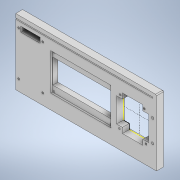
# Autodesk Inventor part: 2020-04-12 CubeBaseFull
Saved by Autodesk Inventor 2020 (Build 240168000, 168)
## iProperties
Created: 2019-12-01
Part Number: 2020-04-12 CubeBaseFull
Material: Generic
Document SubType Name: Modeling
Designer: torto
Density: 1 g/cm^3
Appearance: Default
length: 230.251 mm
height: 107.950 mm
d3: 6.350 mm
d4: 6.350 mm
d5: 223.901 mm
d6: 1.524 mm
spacing: 35.983 mm
d9: 6.350 mm
d10: 3.500 mm
d11: 2.000 ul
d13: 35.983 mm
thickness: 12.700 mm
d19: 0.00 deg
d21: 6.350 mm
d22: 6.350 mm
d23: 223.901 mm
d24: 1.524 mm
d25: 6.350 mm
d26: 0.00 deg
d33: 6.350 mm
d34: 35.983 mm
ScrewDiameter: 4.000 mm
d36: 6.350 mm
d37: 35.983 mm
d38: 4.000 mm
d39: 12.700 mm
d40: 0.00 deg
d49: 106.626 mm
d50: 53.975 mm
LcdLength: 97.300 mm
LcdHeight: 39.800 mm
LcdBorderHeight: 60.200 mm
LcdBorderLength: 98.300 mm
d66: 9.900 mm
d67: 0.00 deg
LcdPcbThickness: 2.800 mm
d69: 0.00 deg
LcdFrameHoleOffset: 2.500 mm
d71: 2.500 mm
LcdFrameHoleDiameter: 3.000 mm
LcdScrewDepth: 6.000 mm
d74: 0.00 deg
InputHeight: 57.400 mm
InputLength: 52.500 mm
InputThickness: 1.600 mm
d78: 0.00 deg
InputHoleSpacing: 0.172 in
d80: 0.278 in
InputScrewDiameter: 3.500 mm
d82: 14.100 mm
d83: 8.500 mm
d84: 11.100 mm
d85: 0.00 deg
InputHoleSpacingX: 7.100 mm
InputHoleSpacingY: 4.250 mm
ScrewDiameterUntapped: 4.000 mm
ScrewCapDiameter: 3.500 mm
PcbThickness: 1.651 mm
TopScrewDiameter: 4.000 mm
InputScrewDiameterUntapped: 2.500 mm
InputScrewDiameterFull: 3.500 mm
InputCornerLengthX: 9.500 mm
InputCornerLengthY: 8.700 mm
UpperInputHoleSpacingY: 4.350 mm
LeftInputHoleSpacingX: 7.100 mm
NWInputHoleSpacingX: 7.250 mm
LcdFrameHoleDiameterUntapped: 2.500 mm
Author: torto
Autodesk Inventor part; units mm, degrees
ref_plane "YZ Plane" through (0, 0, 0) normal (1, 0, 0) x (0, 1, 0)
ref_plane "XZ Plane" through (0, 0, 0) normal (0, 1, 0) x (-1, 0, 0)
ref_plane "XY Plane" through (0, 0, 0) normal (0, 0, 1) x (1, 0, 0)
sketch "Sketch1" plane through (0, 0, 0) normal (0, 0, 1) x (1, 0, 0)
  line L0 (0, 0) -> (230.251, 0)
  line L1 (230.251, 0) -> (230.251, 107.95)
  line L2 (230.251, 107.95) -> (0, 107.95)
  line L3 (0, 107.95) -> (0, 0)
  line L4 (230.251, 107.95) -> (223.901, 107.95) construction
  line L5 (223.901, 107.95) -> (223.901, 101.6) construction
  line L6 (223.901, 101.6) -> (230.251, 101.6) construction
  line L7 (230.251, 101.6) -> (230.251, 107.95) construction
  line L8 (223.901, 101.6) -> (0, 101.6)
  line L9 (0, 101.6) -> (0, 100.076)
  line L10 (0, 100.076) -> (223.901, 100.076)
  line L11 (223.901, 100.076) -> (223.901, 101.6)
  line L12 (230.251, 0) -> (223.901, 0) construction
  line L13 (223.901, 0) -> (223.901, 35.9833) construction
  line L14 (223.901, 35.9833) -> (230.251, 35.9833) construction
  line L15 (230.251, 35.9833) -> (230.251, 0) construction
  circle A0 centre (223.901, 35.9833) radius 2
  circle A1 centre (223.901, 71.9667) radius 2
  dimension "length" = 230.251
  dimension "height" = 107.95
  dimension "d3" = 6.35
  dimension "d4" = 6.35
  dimension "d5" = 223.901
  dimension "d6" = 1.524
  dimension "spacing" = 35.9833
  dimension "d9" = 6.35
  dimension "TopScrewDiameter" = 4
  dimension "d13" = 35.9833
  constraints: 32 end point, 8 parallel, 4 horizontal, 4 perpendicular, 2 centre point, 2 coincident, 1 vertical, 3 other
  measures "length" distance of L2.end L1.end
  measures "height" distance of L1.end L0.end
  measures "d3" distance of L5.end L4.end
  measures "d4" distance of L5.end L6.end
  measures "d5" distance of L10.end L9.end
  measures "d6" distance of L9.end L8.end
  measures "spacing" distance of L12.end L13.end
  measures "d9" distance of L13.end L14.end
  measures "TopScrewDiameter" diameter of A0
  measures "d13" distance of A0.centre A1.centre
extrude "Generic Shape" add sketch "Sketch1" along normal blind 12.7
chamfer "Chamfer Outside Edges" distance 1.5 angle 45 3 edges at (115.1255, 107.95, 0) (230.251, 107.95, 6.35) (230.251, 53.975, 0)
sketch "ScrewCapDiameter" plane through (0, 0, 0) normal (0, 0, -1) x (-1, 0, 0)
  circle A0 centre (-223.901, 71.9667) radius 2 projected
  circle A1 centre (-223.901, 71.9667) radius 4
  circle A2 centre (-223.901, 35.9833) radius 2 projected
  circle A3 centre (-223.901, 35.9833) radius 4
  point P0 (0, 0)
  dimension "d106" = 8
  dimension "d107" = 8
  constraints: 2 centre point, 2 coincident
  measures "d106" diameter of A1
  measures "d107" diameter of A3
extrude "ScrewCapCountersink" cut sketch "ScrewCapDiameter" against normal blind 4
sketch "PcbNotchDimensions" plane through (0, 0, 12.7) normal (0, 0, 1) x (1, 0, 0)
  line L0 (230.251, 107.95) -> (0, 107.95) construction
  line L1 (230.251, 107.95) -> (223.901, 107.95) construction
  line L2 (223.901, 107.95) -> (223.901, 101.6) construction
  line L3 (223.901, 101.6) -> (230.251, 101.6) construction
  line L4 (230.251, 101.6) -> (230.251, 107.95) construction
  line L5 (223.901, 101.6) -> (0, 101.6)
  line L6 (0, 101.6) -> (0, 99.949)
  line L7 (0, 99.949) -> (223.901, 99.949)
  line L8 (223.901, 99.949) -> (223.901, 101.6)
  point P0 (0, 0)
  dimension "d21" = 6.35
  dimension "d22" = 6.35
  dimension "d23" = 223.901
  dimension "PcbThickness" = 1.651
  constraints: 16 end point, 4 parallel, 2 horizontal, 2 perpendicular
  measures "d21" distance of L2.end L1.end
  measures "d22" distance of L2.end L3.end
  measures "d23" distance of L7.end L6.end
  measures "PcbThickness" distance of L6.end L5.end
extrude "PCB Notch" cut sketch "PcbNotchDimensions" against normal blind 6.35
sketch "UntappedScrewHoleDimensions" plane through (0, 0, 0) normal (-1, 0, 0) x (0, 0, 1)
  line L0 (0, 0) -> (6.35, 0) construction
  line L1 (6.35, 0) -> (6.35, 35.9833) construction
  line L2 (6.35, 35.9833) -> (0, 35.9833) construction
  line L3 (0, 35.9833) -> (0, 0) construction
  circle A0 centre (6.35, 35.9833) radius 2
  line L4 (0, 107.95) -> (6.35, 107.95) construction
  line L5 (6.35, 107.95) -> (6.35, 71.9667) construction
  line L6 (6.35, 71.9667) -> (0, 71.9667) construction
  line L7 (0, 71.9667) -> (0, 107.95) construction
  circle A1 centre (6.35, 71.9667) radius 2
  dimension "d33" = 6.35
  dimension "d34" = 35.9833
  dimension "ScrewDiameterUntapped" = 4
  dimension "d36" = 6.35
  dimension "d37" = 35.9833
  dimension "d38" = 4
  constraints: 16 end point, 4 parallel, 2 centre point, 2 coincident, 2 horizontal, 2 perpendicular
  measures "d33" distance of L2.end L1.end
  measures "d34" distance of L1.end L0.end
  measures "ScrewDiameterUntapped" diameter of A0
  measures "d36" distance of L5.end L6.end
  measures "d37" distance of L4.end L5.end
  measures "d38" diameter of A1
extrude "UntappedScrewDepth" cut sketch "UntappedScrewHoleDimensions" against normal blind 12.7
sketch "LCD" plane through (0, 0, 0) normal (0, 0, -1) x (-1, 0, 0)
  line L0 (0, 0) -> (-230.251, 0) construction
  line L1 (0, 0) -> (-106.6255, 0) construction
  line L2 (-106.6255, 0) -> (-106.6255, 53.975) construction
  line L3 (-106.6255, 53.975) -> (0, 53.975) construction
  line L4 (0, 53.975) -> (0, 0) construction
  line L5 (-155.2755, 73.875) -> (-57.9755, 73.875)
  line L6 (-57.9755, 73.875) -> (-57.9755, 34.075)
  line L7 (-57.9755, 34.075) -> (-155.2755, 34.075)
  line L8 (-155.2755, 34.075) -> (-155.2755, 73.875)
  line L9 (-155.2755, 73.875) -> (-57.9755, 34.075) construction
  line L10 (-57.9755, 73.875) -> (-155.2755, 34.075) construction
  line L11 (-155.7755, 84.075) -> (-57.4755, 84.075)
  line L12 (-57.4755, 84.075) -> (-57.4755, 23.875)
  line L13 (-57.4755, 23.875) -> (-155.7755, 23.875)
  line L14 (-155.7755, 23.875) -> (-155.7755, 84.075)
  line L15 (-155.7755, 84.075) -> (-57.4755, 23.875) construction
  line L16 (-57.4755, 84.075) -> (-155.7755, 23.875) construction
  dimension "d49" = 106.6255
  dimension "d50" = 53.975
  dimension "LcdLength" = 97.3
  dimension "LcdHeight" = 39.8
  dimension "LcdBorderHeight" = 60.2
  dimension "LcdBorderLength" = 98.3
  constraints: 32 end point, 6 parallel, 4 midpoint, 3 horizontal, 3 perpendicular
  measures "d49" distance of L2.end L3.end
  measures "d50" distance of L1.end L2.end
  measures "LcdLength" distance of L6.end L7.end
  measures "LcdHeight" distance of L7.end L5.start
  measures "LcdBorderHeight" distance of L11.end L12.end
  measures "LcdBorderLength" distance of L12.end L13.end
extrude "LcdWindow" cut sketch "LCD" against normal blind 9.9 contours L5 L6 L7 L8
sketch "LcdFrameDimensions" plane through (0, 0, 12.7) normal (0, 0, 1) x (1, 0, 0)
  line L0 (155.7755, 84.075) -> (57.4755, 84.075) projected
  line L1 (155.7755, 23.875) -> (155.7755, 84.075) projected
  line L2 (57.4755, 23.875) -> (155.7755, 23.875) projected
  line L3 (57.4755, 84.075) -> (57.4755, 23.875) projected
  point P0 (0, 0)
extrude "LcdFrame" cut sketch "LcdFrameDimensions" against normal blind 2.8
sketch "LcdScrewsSketch" plane through (0, 0, 9.9) normal (0, 0, 1) x (1, 0, 0)
  line L0 (57.4755, 23.875) -> (57.4755, 84.075) construction
  line L1 (57.4755, 84.075) -> (59.9755, 84.075) construction
  line L2 (59.9755, 84.075) -> (59.9755, 81.575) construction
  line L3 (59.9755, 81.575) -> (57.4755, 81.575) construction
  line L4 (57.4755, 81.575) -> (57.4755, 84.075) construction
  circle A0 centre (59.9755, 81.575) radius 1.25
  line L5 (57.4755, 84.075) -> (155.7755, 84.075) construction
  line L6 (106.6255, 84.075) -> (106.6255, 23.875) construction
  line L7 (155.7755, 23.875) -> (57.4755, 23.875) construction
  line L8 (57.4755, 53.975) -> (155.7755, 53.975) construction
  line L9 (155.7755, 84.075) -> (155.7755, 23.875) construction
  circle A1 centre (153.2755, 81.575) radius 1.25
  circle A2 centre (59.9755, 26.375) radius 1.25
  circle A3 centre (153.2755, 26.375) radius 1.25
  point P0 (0, 0)
  dimension "LcdFrameHoleOffset" = 2.5
  dimension "d71" = 2.5
  dimension "LcdFrameHoleDiameterUntapped" = 2.5
  constraints: 12 end point, 4 centre point, 4 midpoint, 3 symmetric about line, 2 parallel, 1 coincident, 1 horizontal, 1 perpendicular, 3 other
  measures "LcdFrameHoleOffset" distance of L2.end L3.end
  measures "d71" distance of L1.end L2.end
  measures "LcdFrameHoleDiameterUntapped" diameter of A0
extrude "LcdScrews" cut sketch "LcdScrewsSketch" against normal blind 6
sketch "InputDimensions" plane through (0, 0, 0) normal (0, 0, 1) x (1, 0, 0)
  line L0 (155.2755, 34.075) -> (155.2755, 73.875) construction
  line L1 (230.251, 0) -> (230.251, 107.95) construction
  line L2 (165.051, 82.675) -> (217.551, 82.675)
  line L3 (217.551, 82.675) -> (217.551, 25.275)
  line L4 (217.551, 25.275) -> (165.051, 25.275)
  line L5 (165.051, 25.275) -> (165.051, 82.675)
  line L6 (230.251, 107.95) -> (191.389, 107.95) construction
  line L7 (230.251, 53.975) -> (230.251, 107.95) construction
  line L8 (217.551, 82.675) -> (165.051, 25.275) construction
  line L9 (217.551, 25.275) -> (165.051, 82.675) construction
  line L10 (191.301, 53.975) -> (230.251, 53.975) construction
  line L11 (230.251, 53.975) -> (230.251, 107.95) construction
  line L12 (230.251, 107.95) -> (191.301, 107.95) construction
  line L13 (191.301, 107.95) -> (191.301, 53.975) construction
  point P0 (0, 0)
  dimension "InputHeight" = 57.4
  dimension "InputLength" = 52.5
  dimension "d93" = 38.95
  dimension "d94" = 53.975
  constraints: 24 end point, 4 parallel, 3 horizontal, 2 perpendicular, 1 midpoint
  measures "InputHeight" distance of L4.end L2.start
  measures "InputLength" distance of L3.end L4.end
  measures "d93" distance of L10.start L10.end
  measures "d94" distance of L12.end L10.start
extrude "InputCountersink" cut sketch "InputDimensions" along normal blind 1.6
sketch "InputCorners" plane through (0, 0, 1.6) normal (0, 0, -1) x (-1, 0, 0)
  line L0 (-217.551, 25.275) -> (-217.551, 82.675) projected
  line L1 (-217.551, 82.675) -> (-210.301, 82.675) construction
  line L2 (-210.301, 82.675) -> (-210.301, 78.325) construction
  line L3 (-210.301, 78.325) -> (-217.551, 78.325) construction
  line L4 (-217.551, 78.325) -> (-217.551, 82.675) construction
  circle A0 centre (-210.301, 78.325) radius 1.75 construction
  line L5 (-217.551, 82.675) -> (-165.051, 82.675) projected
  line L6 (-191.301, 82.675) -> (-191.301, 25.275) construction
  line L7 (-165.051, 25.275) -> (-217.551, 25.275) projected
  line L8 (-217.551, 53.975) -> (-165.051, 53.975) construction
  line L9 (-165.051, 82.675) -> (-165.051, 25.275) projected
  line L10 (-217.551, 82.675) -> (-208.051, 82.675) construction
  line L11 (-208.051, 82.675) -> (-208.051, 73.975)
  line L12 (-208.051, 73.975) -> (-217.551, 73.975)
  line L13 (-217.551, 73.975) -> (-217.551, 82.675) construction
  line L14 (-174.551, 82.675) -> (-174.551, 73.975)
  line L15 (-174.551, 73.975) -> (-165.051, 73.975)
  line L16 (-208.051, 25.275) -> (-208.051, 33.975)
  line L17 (-208.051, 33.975) -> (-217.551, 33.975)
  line L18 (-174.551, 33.975) -> (-165.051, 33.975)
  line L19 (-174.551, 25.275) -> (-174.551, 33.975)
  circle A1 centre (-210.301, 78.325) radius 1.5
  line L20 (-165.051, 82.675) -> (-170.901, 82.675) construction
  line L21 (-170.901, 82.675) -> (-170.901, 78.325) construction
  line L22 (-170.901, 78.325) -> (-165.051, 78.325) construction
  line L23 (-165.051, 78.325) -> (-165.051, 82.675) construction
  line L24 (-217.551, 25.275) -> (-213.101, 25.275) construction
  line L25 (-213.101, 25.275) -> (-213.101, 29.725) construction
  line L26 (-213.101, 29.725) -> (-217.551, 29.725) construction
  line L27 (-217.551, 29.725) -> (-217.551, 25.275) construction
  line L28 (-165.051, 25.275) -> (-169.501, 25.275) construction
  line L29 (-169.501, 25.275) -> (-169.501, 29.725) construction
  line L30 (-169.501, 29.725) -> (-165.051, 29.725) construction
  line L31 (-165.051, 29.725) -> (-165.051, 25.275) construction
  circle A2 centre (-213.101, 29.725) radius 1.5
  circle A3 centre (-169.501, 29.725) radius 1.5
  line L32 (-165.051, 82.675) -> (-165.051, 25.275) projected
  circle A4 centre (-170.901, 78.325) radius 1.5
  point P0 (0, 0)
  point P1 (-174.551, 82.675)
  point P2 (-208.051, 82.675)
  point P3 (-208.051, 25.275)
  point P4 (-174.551, 25.275)
  dimension "NWInputHoleSpacingX" = 7.25
  dimension "UpperInputHoleSpacingY" = 4.35
  dimension "InputScrewDiameterFull" = 3.5
  dimension "InputCornerLengthX" = 9.5
  dimension "InputCornerLengthY" = 8.7
  dimension "InputScrewDiameterUntapped" = 3
  dimension "NEInputHoleSpacingX" = 5.85
  dimension "d134" = 4.35
  dimension "LowerInputHoleSpacingY" = 4.45
  dimension "SWInputHoleSpacingX" = 4.45
  dimension "d138" = 4.45
  dimension "SEInputHoleSpacingX" = 4.45
  dimension "d140" = 3
  dimension "d141" = 3
  dimension "d142" = 3
  constraints: 56 end point, 10 parallel, 9 symmetric about line, 5 centre point, 5 coincident, 5 horizontal, 5 perpendicular, 4 midpoint, 1 collinear, 1 point on line
  measures "NWInputHoleSpacingX" distance of L2.end L3.end
  measures "UpperInputHoleSpacingY" distance of L1.end L2.end
  measures "InputScrewDiameterFull" diameter of A0
  measures "InputCornerLengthX" distance of L11.end L12.end
  measures "InputCornerLengthY" distance of L10.end L11.end
  measures "InputScrewDiameterUntapped" diameter of A1
  measures "NEInputHoleSpacingX" distance of L22.end L21.end
  measures "d134" distance of L20.end L21.end
  measures "LowerInputHoleSpacingY" distance of L25.end L24.end
  measures "SWInputHoleSpacingX" distance of L25.end L26.end
  measures "d138" distance of L28.end L29.end
  measures "SEInputHoleSpacingX" distance of L29.end L30.end
  measures "d140" diameter of A2
  measures "d141" diameter of A3
  measures "d142" diameter of A4
extrude "InputCut" cut sketch "InputCorners" against normal blind 11.1 contours L0 L12 L11 L5 L14 L15 L9 L18 L19 L7 L16 L17 | A1 | A2 | A3 | A4
chamfer "LcdChamfer" distance 1.651 angle 45 4 edges at (106.6255, 73.875, 0) (155.2755, 53.975, 0) (106.6255, 34.075, 0) (57.9755, 53.975, 0)
sketch "KeypadDimensions" plane through (0, 0, 0) normal (0, 0, -1) x (-1, 0, 0)
  line L0 (-48.3, 94.175) -> (0, 94.175)
  line L1 (0, 94.175) -> (0, 13.775)
  line L2 (0, 13.775) -> (-48.3, 13.775)
  line L3 (-48.3, 13.775) -> (-48.3, 94.175)
  line L4 (-48.3, 94.175) -> (0, 13.775) construction
  line L5 (-48.3, 13.775) -> (0, 94.175) construction
  line L6 (0, 107.95) -> (0, 0) construction
  line L7 (0, 0) -> (-24.15, 0) construction
  line L8 (-24.15, 0) -> (-24.15, 53.975) construction
  line L9 (-24.15, 53.975) -> (0, 53.975) construction
  line L10 (0, 53.975) -> (0, 0) construction
  point P0 (0, 99.949)
  dimension "KeypadLength" = 48.3
  dimension "KeypadHeight" = 80.4
  dimension "d97" = 53.975
  dimension "d98" = 24.15
  constraints: 20 end point, 4 parallel, 2 horizontal, 2 perpendicular, 1 midpoint
  measures "KeypadLength" distance of L0.start L0.end
  measures "KeypadHeight" distance of L2.end L0.start
  measures "d97" distance of L7.end L8.end
  measures "d98" distance of L8.end L9.end
extrude "KeypadCountersink" cut sketch "KeypadDimensions" against normal blind 2
sketch "KeypadCorners" plane through (0, 0, 2) normal (0, 0, -1) x (-1, 0, 0)
  line L0 (-48.3, 13.775) -> (-48.3, 94.175) construction
  line L1 (-48.3, 94.175) -> (-44.35, 94.175) construction
  line L2 (-44.35, 94.175) -> (-44.35, 89.925) construction
  line L3 (-44.35, 89.925) -> (-48.3, 89.925) construction
  line L4 (-48.3, 89.925) -> (-48.3, 94.175) construction
  circle A0 centre (-44.35, 89.925) radius 1.75 construction
  circle A1 centre (-44.35, 89.925) radius 1.5
  line L5 (-48.3, 94.175) -> (-39.8, 94.175)
  line L6 (-39.8, 94.175) -> (-39.8, 85.675)
  line L7 (-39.8, 85.675) -> (-48.3, 85.675)
  line L8 (-48.3, 85.675) -> (-48.3, 94.175)
  line L9 (-48.3, 94.175) -> (0, 94.175) construction
  line L10 (-24.15, 94.175) -> (-24.15, 13.775) construction
  line L11 (0, 13.775) -> (-48.3, 13.775) construction
  line L12 (-48.3, 53.975) -> (0, 53.975) construction
  line L13 (0, 107.95) -> (0, 0) construction
  line L14 (-8.5, 94.175) -> (-8.5, 85.675)
  line L15 (-8.5, 85.675) -> (0, 85.675)
  line L16 (-39.8, 13.775) -> (-39.8, 22.275)
  line L17 (-39.8, 22.275) -> (-48.3, 22.275)
  line L18 (-8.5, 22.275) -> (0, 22.275)
  line L19 (-8.5, 13.775) -> (-8.5, 22.275)
  line L20 (-39.8, 85.675) -> (-8.5, 85.675)
  line L21 (0, 94.175) -> (-4.95, 94.175) construction
  line L22 (-4.95, 94.175) -> (-4.95, 89.925) construction
  line L23 (-4.95, 89.925) -> (0, 89.925) construction
  line L24 (0, 89.925) -> (0, 94.175) construction
  line L25 (0, 13.775) -> (-4.95, 13.775) construction
  line L26 (-4.95, 13.775) -> (-4.95, 17.725) construction
  line L27 (-4.95, 17.725) -> (0, 17.725) construction
  line L28 (0, 17.725) -> (0, 13.775) construction
  circle A2 centre (-4.95, 17.725) radius 1.5
  line L29 (-48.3, 13.775) -> (-44.35, 13.775) construction
  line L30 (-44.35, 13.775) -> (-44.35, 17.725) construction
  line L31 (-44.35, 17.725) -> (-48.3, 17.725) construction
  line L32 (-48.3, 17.725) -> (-48.3, 13.775) construction
  circle A3 centre (-44.35, 17.725) radius 1.5
  circle A4 centre (-4.95, 89.925) radius 1.5
  line L33 (-39.8, 94.175) -> (-8.5, 94.175)
  point P0 (0, 99.949)
  dimension "LeftKeypadHoleSpacingX" = 3.95
  dimension "UpperKeypadHoleSpacingY" = 4.25
  dimension "KeypadHoleDiameter" = 3.5
  dimension "KeypadScrewHoleDiameterUntapped" = 3
  dimension "KeypadCornerLengthX" = 8.5
  dimension "KeypadCornerLengthY" = 8.5
  dimension "RightKeypadHoleSpacingX" = 4.95
  dimension "d118" = 4.25
  dimension "d121" = 4.95
  dimension "LowerKeypadHoleSpacingY" = 3.95
  dimension "d123" = 3
  dimension "d124" = 3.95
  dimension "d125" = 3.95
  dimension "d126" = 3
  dimension "d127" = 3
  constraints: 60 end point, 10 parallel, 9 symmetric about line, 6 horizontal, 6 perpendicular, 5 centre point, 5 coincident, 4 midpoint, 1 collinear
  measures "LeftKeypadHoleSpacingX" distance of L2.end L3.end
  measures "UpperKeypadHoleSpacingY" distance of L1.end L2.end
  measures "KeypadHoleDiameter" diameter of A0
  measures "KeypadScrewHoleDiameterUntapped" diameter of A1
  measures "KeypadCornerLengthX" distance of L6.end L7.end
  measures "KeypadCornerLengthY" distance of L5.end L6.end
  measures "RightKeypadHoleSpacingX" distance of L23.end L22.end
  measures "d118" distance of L22.end L21.end
  measures "d121" distance of L26.end L27.end
  measures "LowerKeypadHoleSpacingY" distance of L25.end L26.end
  measures "d123" diameter of A2
  measures "d124" distance of L31.end L30.end
  measures "d125" distance of L29.end L30.end
  measures "d126" diameter of A3
  measures "d127" diameter of A4
extrude "KeypadHoles" cut sketch "KeypadCorners" against normal blind 11.1 contours A1 | L33 L14 L20 L6 | A2 | A3 | A4
thread "KeypadThreadNW" size "M3x0.5" class "6H" standard "ANSI Metric M Profile" full length
thread "KeypadThreadNE" size "M3x0.5" class "6H" standard "ANSI Metric M Profile" full length
thread "KeypadThreadSW" size "M3x0.5" class "6H" standard "ANSI Metric M Profile" full length
thread "KeypadThreadSE" size "M3x0.5" class "6H" standard "ANSI Metric M Profile" full length
thread "SideThreadTop" size "M4x0.7" class "6H" standard "ANSI Metric M Profile" length 230.251
thread "SideThreadBottom" size "M4x0.7" class "6H" standard "ANSI Metric M Profile" length 230.251
thread "InputThreadNW" size "M3x0.5" class "6H" standard "ANSI Metric M Profile" length 12.7
thread "InputThreadNE" size "M3x0.5" class "6H" standard "ANSI Metric M Profile" length 12.7
thread "InputThreadSE" size "M3x0.5" class "6H" standard "ANSI Metric M Profile" length 12.7
thread "InputThreadSW" size "M3x0.5" class "6H" standard "ANSI Metric M Profile" length 12.7
equation "\"d3\" = 0.5 * thickness"
equation "\"d4\" = 0.5 * thickness"
equation "\"d5\" = length - 0.5 * thickness"
equation "\"spacing\" = 0.333333 * height"
equation "\"d9\" = 0.5 * thickness"
equation "\"d13\" = spacing"
equation "\"d25\" = 0.5 * thickness"
equation "\"d33\" = 0.5 * thickness"
equation "\"d34\" = 0.333333 * height"
equation "\"d36\" = 0.5 * thickness"
equation "\"d37\" = 0.333333 * height"
equation "\"d38\" = ScrewDiameterUntapped"
equation "\"d50\" = 0.5 * height"
equation "\"d66\" = thickness - LcdPcbThickness"
equation "\"LcdPcbThickness\" = thickness - LcdThickness"
equation "\"d71\" = LcdFrameHoleOffset"
equation "\"d93\" = thickness + 0.5 * InputLength"
equation "\"d94\" = 0.5 * height"
equation "\"d84\" = thickness - InputThickness"
equation "\"d97\" = 0.5 * height"
equation "\"d98\" = 0.5 * KeypadLength"
equation "\"LcdThickness\" = 9.9"
equation "\"thickness\" = 12.7"
equation "\"InputThickness\" = 1.6"
body "Solid1"
